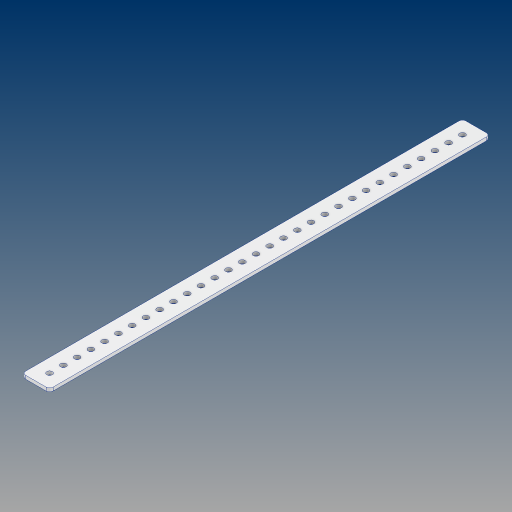
# Autodesk Inventor part: ELEV_016_SUPBAR1
Saved by Autodesk Inventor 2024.3 (Build 283343000, 343)
## iProperties
Created: 2024-11-27
Part Number: ELEV_016_SUPBAR1
Material: Aluminum 6061
Document SubType Name: Modeling
Designer: Kenji
Mass: 83.0297 g
Surface Area: 236.666 cm^2
Volume: 30.7517 cm^3
Density: 2.7 g/cm^3
Appearance: Aluminum - Flat
Author: Kenji
Autodesk Inventor part; units mm, degrees
ref_plane "YZ Plane" through (0, 0, 0) normal (1, 0, 0) x (0, 1, 0)
ref_plane "XZ Plane" through (0, 0, 0) normal (0, 1, 0) x (-1, 0, 0)
ref_plane "XY Plane" through (0, 0, 0) normal (0, 0, 1) x (1, 0, 0)
sketch "Sketch1" plane through (0, 0, 0) normal (0, 1, 0) x (-1, 0, 0)
  line L0 (3.175, 0) -> (22.225, 0)
  line L1 (25.4, -3.175) -> (25.4, -403.225)
  line L2 (22.225, -406.4) -> (3.175, -406.4)
  line L3 (0, -403.225) -> (0, -3.175)
  arc A0 (25.4, -3.175) -> (22.225, 0) centre (22.225, -3.175) ccw
  arc A1 (3.175, 0) -> (0, -3.175) centre (3.175, -3.175) ccw
  arc A2 (22.225, -406.4) -> (25.4, -403.225) centre (22.225, -403.225) ccw
  arc A3 (0, -403.225) -> (3.175, -406.4) centre (3.175, -403.225) ccw
  circle A4 centre (12.7, -12.7) radius 2.54
  circle A5 centre (12.7, -25.4) radius 2.54
  circle A6 centre (12.7, -38.1) radius 2.54
  circle A7 centre (12.7, -50.8) radius 2.54
  circle A8 centre (12.7, -63.5) radius 2.54
  circle A9 centre (12.7, -76.2) radius 2.54
  circle A10 centre (12.7, -88.9) radius 2.54
  circle A11 centre (12.7, -101.6) radius 2.54
  circle A12 centre (12.7, -114.3) radius 2.54
  circle A13 centre (12.7, -127) radius 2.54
  circle A14 centre (12.7, -139.7) radius 2.54
  circle A15 centre (12.7, -152.4) radius 2.54
  circle A16 centre (12.7, -165.1) radius 2.54
  circle A17 centre (12.7, -177.8) radius 2.54
  circle A18 centre (12.7, -190.5) radius 2.54
  circle A19 centre (12.7, -203.2) radius 2.54
  circle A20 centre (12.7, -215.9) radius 2.54
  circle A21 centre (12.7, -228.6) radius 2.54
  circle A22 centre (12.7, -241.3) radius 2.54
  circle A23 centre (12.7, -254) radius 2.54
  circle A24 centre (12.7, -266.7) radius 2.54
  circle A25 centre (12.7, -279.4) radius 2.54
  circle A26 centre (12.7, -292.1) radius 2.54
  circle A27 centre (12.7, -304.8) radius 2.54
  circle A28 centre (12.7, -317.5) radius 2.54
  circle A29 centre (12.7, -330.2) radius 2.54
  circle A30 centre (12.7, -342.9) radius 2.54
  circle A31 centre (12.7, -355.6) radius 2.54
  circle A32 centre (12.7, -368.3) radius 2.54
  circle A33 centre (12.7, -381) radius 2.54
  circle A34 centre (12.7, -393.7) radius 2.54
  point P0 (0, 0)
  dimension "d0" = 25.4
  dimension "d1" = 406.4
  dimension "d2" = 3.175
  dimension "d3" = 3.175
  dimension "d4" = 12.7
  dimension "d5" = 5.08
  dimension "d6" = 12.7
  dimension "d9" = 12.7
  constraints: 35 centre point, 8 end point, 8 point on circle, 8 tangent, 2 equal radius, 2 parallel, 2 point on line, 1 horizontal, 1 perpendicular, 1 vertical, 60 other
  measures "d0" distance between parallel lines of L3 L1
  measures "d1" distance between parallel lines of L2 L0
  measures "d2" radius of A0
  measures "d3" radius of A1
  measures "d4" distance from line of L0 A4.centre
  measures "d5" diameter of A4
  measures "d6" distance from line of L1 A4.centre
  measures "d9" distance of A4.centre A5.centre
extrude "Extrusion1" add sketch "Sketch1" along normal blind 3.175
body "Solid1"
